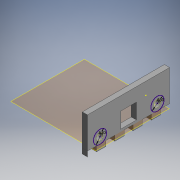
# Autodesk Inventor part: Part15
Saved by Autodesk Inventor 2016 (Build 200138000, 138)
## iProperties
Created: 2018-01-18
Part Number: Part15
Material: Generic
Document SubType Name: Modeling
Designer: student
Density: 1 g/cm^3
Appearance: Default
Author: student
Autodesk Inventor part; units mm, degrees
ref_plane "YZ Plane" through (0, 0, 0) normal (1, 0, 0) x (0, 1, 0)
ref_plane "XZ Plane" through (0, 0, 0) normal (0, 1, 0) x (-1, 0, 0)
ref_plane "XY Plane" through (0, 0, 0) normal (0, 0, 1) x (1, 0, 0)
ref_plane "Work Plane1" through (-108.8053, -23.2276, 20.9918) normal (0, 1, 0) x (-0.9999918, 0, -0.00406)
sketch "Sketch1" plane through (-108.8053, -23.2276, 20.9918) normal (0, 1, 0) x (-0.9999918, 0, -0.00406)
  line L0 (-46.787, -50.1863) -> (-47.193, 49.8137)
  line L1 (-47.193, 49.8137) -> (-40.843, 49.8137)
  line L2 (-46.787, -50.1863) -> (-40.437, -50.1863)
  line L3 (-46.787, -50.1863) -> (-40.437, -50.1863)
  line L4 (-40.843, 49.8137) -> (-40.437, -50.1863)
  line L5 (-47.193, 49.8137) -> (46.787, 50.1953) construction
  point P0 (-108.7192, -21.4334)
  dimension "d0" = 6.35
  dimension "d1" = 6.35
  constraints: 10 end point, 3 horizontal, 1 coincident, 1 collinear
  measures "d0" distance of L0.end L1.end
  measures "d1" distance of L0.start L2.end
extrude "Extrusion1" add sketch "Sketch1" along normal blind 38.1 and the other way blind 6.35
sketch "Sketch2" plane through (-61.8149, -29.5776, 70.9967) normal (1, 0, 0) x (0, 0, -1)
  line L0 (100.0008, 0) -> (0, 0) construction
  line L1 (100.0008, 0) -> (100.0008, 44.45) construction
  line L2 (0, 44.45) -> (100.0008, 44.45) construction
  line L3 (0, 0) -> (0, 44.45) construction
  line L4 (0, 44.45) -> (100.0008, 44.45) construction
  line L5 (50.0004, 44.45) -> (50.0004, 0) construction
  circle A0 centre (15.0004, 13.9978) radius 4
  circle A1 centre (85.0004, 13.9978) radius 4
  line L6 (40.4004, 9.271) -> (59.6004, 9.271)
  line L7 (59.6004, 9.271) -> (59.6004, 28.291)
  line L8 (59.6004, 28.291) -> (40.4004, 28.291)
  line L9 (40.4004, 28.291) -> (40.4004, 9.271)
  line L10 (21.3504, 9.271) -> (21.3504, 25.4) construction
  line L11 (21.3504, 20.3478) -> (13.3504, 20.3478) construction
  line L12 (21.3504, 9.271) -> (21.3504, 25.4) projected
  line L13 (78.6504, 9.271) -> (78.6504, 25.4) projected
  line L14 (11.1112, 0) -> (11.1112, 6.35) projected
  line L15 (22.2224, 6.35) -> (22.2224, 0) projected
  line L16 (33.3334, 0) -> (33.3334, 6.35) projected
  line L17 (44.4446, 6.35) -> (44.4446, 0) projected
  line L18 (55.5556, 0) -> (55.5556, 6.35) projected
  line L19 (66.6668, 6.35) -> (66.6668, 0) projected
  line L20 (88.8891, 6.35) -> (88.8891, 0) projected
  line L21 (77.7779, 0) -> (77.7779, 6.35) projected
  line L22 (88.8891, 6.35) -> (100.0008, 6.35) construction
  line L23 (100.0008, 0) -> (88.8891, 0) construction
  line L24 (0.0258, 0) -> (100.0266, 0) construction
  line L25 (66.6668, 0) -> (77.7779, 0) construction
  line L26 (55.5556, 0) -> (44.4446, 0) construction
  line L27 (33.3334, 0) -> (22.2224, 0) construction
  line L28 (11.1112, 0) -> (0.0258, 0) construction
  line L29 (0.0258, 0) -> (0.0258, 6.35) construction
  line L30 (0.0258, 44.45) -> (0.0258, 0) construction
  line L31 (88.8891, 0) -> (100.0266, 0)
  line L32 (100.0008, 6.35) -> (88.8891, 6.35)
  line L33 (77.7779, 0) -> (66.6668, 0)
  line L34 (66.6668, 6.35) -> (77.7779, 6.35)
  line L35 (55.5556, 0) -> (44.4446, 0)
  line L36 (44.4446, 6.35) -> (55.5556, 6.35)
  line L37 (33.3334, 0) -> (22.2224, 0)
  line L38 (22.2224, 6.35) -> (33.3334, 6.35)
  line L39 (11.1112, 0) -> (0.0258, 0)
  line L40 (11.1112, 6.35) -> (0.0258, 6.35)
  line L41 (0.0258, 0) -> (0.0258, 6.35)
  line L42 (100.0266, 0) -> (100.0008, 6.35)
  line L43 (59.6004, 9.271) -> (59.6004, 25.4) projected
  line L44 (40.4004, 9.271) -> (40.4004, 25.4) projected
  point P0 (70.9967, 23.2276)
  point P1 (75.0381, 0)
  dimension "d9" = 8
  dimension "d10" = 8
  dimension "d13" = 35
  dimension "d14" = 8
  constraints: 52 end point, 11 horizontal, 6 parallel, 4 perpendicular, 4 point on line, 2 centre point, 1 coincident, 1 collinear, 1 midpoint, 1 symmetric about line, 3 other
  measures "d9" diameter of A0
  measures "d10" diameter of A1
  measures "d13" distance from line of L5 A0.centre
  measures "d14" distance of L11.start L11.end
extrude "Extrusion2" cut sketch "Sketch2" against normal blind 35
sketch "Sketch3" plane through (-61.8149, -29.5776, 70.9967) normal (1, 0, 0) x (0, 0, -1)
  circle A0 centre (15.0004, 13.9978) radius 4 construction
  circle A1 centre (85.0004, 13.9978) radius 4 construction
  circle A2 centre (15.0004, 13.9978) radius 8
  circle A3 centre (85.0004, 13.9978) radius 8
  point P0 (70.9967, 29.5776)
  dimension "d22" = 16
  dimension "d23" = 16
  constraints: 2 centre point, 2 coincident
  measures "d22" diameter of A2
  measures "d23" diameter of A3
equation "\"d11\" = d13"
body "Solid1"
